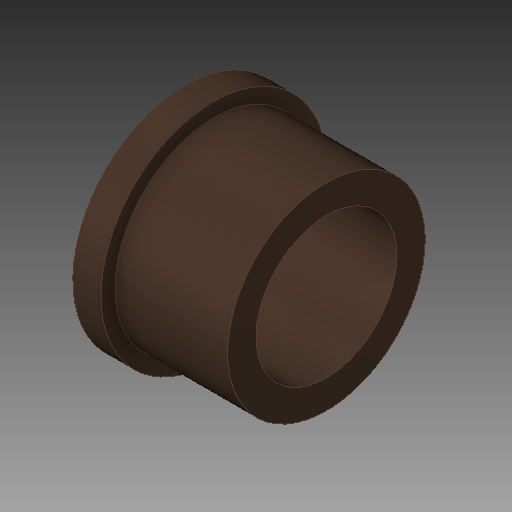
# Autodesk Inventor part: Buje de la Flecha
Saved by Autodesk Inventor 2020 (Build 240168000, 168)
## iProperties
Created: 2016-04-28
Part Number: Buje de la Flecha
Material: Bronze, Cast
Document SubType Name: Modeling
Designer: Jorge
Density: 8.87 g/cm^3
Appearance: Bronze - Satin
Mass: 30.2508 g
Surface Area: 25.5089 cm^2
Volume: 3.41046 cm^3
Author: Jorge
Autodesk Inventor part; units mm, degrees
ref_plane "YZ Plane" through (0, 0, 0) normal (1, 0, 0) x (0, 1, 0)
ref_plane "XZ Plane" through (0, 0, 0) normal (0, 1, 0) x (-1, 0, 0)
ref_plane "XY Plane" through (0, 0, 0) normal (0, 0, 1) x (1, 0, 0)
sketch "Sketch1" plane through (0, 0, 0) normal (0, 0, 1) x (1, 0, 0)
  line L0 (0, 12.7) -> (3.175, 12.7)
  line L1 (3.175, 12.7) -> (3.175, 11.1315)
  line L2 (3.175, 11.1315) -> (15.875, 11.1315)
  line L3 (15.875, 11.1315) -> (15.875, 7.9375)
  line L4 (15.875, 7.9375) -> (0, 7.9375)
  line L5 (0, 7.9375) -> (0, 12.7)
  line L6 (-3.175, 0) -> (19.05, 0) projected
  point P0 (0, 0)
  dimension "d1" = 15.875
  dimension "d2" = 22.2631
  dimension "d3" = 25.4
  dimension "d7" = 15.875
  dimension "d10" = 3.175
  constraints: 12 end point, 5 perpendicular, 1 horizontal
  measures "d1" diameter of L4 L6
  measures "d2" diameter of L2 L6
  measures "d3" diameter of L0 L6
  measures "d7" distance between parallel lines of L3 L5
  measures "d10" distance between parallel lines of L5 L1
revolve "Revolution1" add sketch "Sketch1" angle 360 about axis through (-10, 0, 0) along (1, 0, 0)
body "Solid1"
